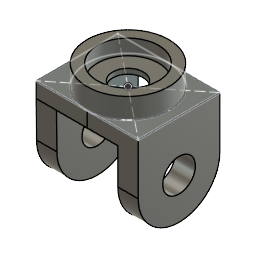
d2 (Autodesk Fusion 360 design; units mm, degrees)
part number: 2026-08-20-16-30-49-448
Autodesk Fusion 360 part; units mm, degrees
sketch "Sketch1" plane through (0, 0, 0) normal (0, 1, 0) x (1, 0, 0)
  line L0 (50, 40) -> (-50, 40)
  line L1 (-50, 40) -> (-50, -40)
  line L2 (-50, -40) -> (50, -40)
  line L3 (50, -40) -> (50, 40)
  line L4 (50, 40) -> (-50, -40) construction
  line L5 (-50, 40) -> (50, -40) construction
  circle A0 centre (0, 0) radius 40
  dimension "d1" = 100
  dimension "d2" = 80
  constraint horizontal L0
  constraint perpendicular L0 L1
  constraint parallel L0 L2
  constraint parallel L1 L3
  constraint coincident L4 A0.centre
  constraint coincident L5 A0.centre
  constraint coincident A0.centre origin
  constraint tangent L0 A0
  measures "d1" distance of L1.end L2.end
  measures "d2" distance of L0.end L1.end
extrude "Extrude1" add sketch "Sketch1" against normal blind 15 contours L0 L2 L3 A0 | L0 L1 L2 A0 makes body 1 at (-3.9827, -10, 39.8012)
extrude "Extrude2" add sketch "Sketch1" along normal blind 20 separate body contours A0 makes body 2
sketch "Sketch2" plane through (0, 20, 0) normal (0, 1, 0) x (-1, 0, 0)
  circle A0 centre (0, 0) radius 40
  circle A1 centre (0, 0) radius 30
  dimension "d7" = 60
  constraint concentric A0 A1
  measures "d7" diameter of A1
extrude "Extrude3" cut sketch "Sketch2" against normal blind 15 contours A1 bodies 2
sketch "Sketch3" plane through (0, 5, 0) normal (0, 1, 0) x (-1, 0, 0)
  circle A0 centre (0, 0) radius 30
  circle A1 centre (0, 0) radius 15
  dimension "d10" = 30
  constraint coincident A0.centre A1.centre
  measures "d10" diameter of A1
extrude "Extrude4" cut sketch "Sketch3" against normal blind 20 contours A1 bodies 2
sketch "Sketch4" plane through (50, 0, 0) normal (1, 0, 0) x (0, 0, -1)
  line L0 (40, 0) -> (-40, 0)
  line L1 (-40, 0) -> (-40, -15)
  line L2 (-40, -15) -> (40, -15)
  line L3 (40, -15) -> (40, 0)
  line L4 (40, -15) -> (40, -50)
  line L5 (-40, -50) -> (-40, -15)
  circle A0 centre (0, -50) radius 16
  arc A1 (-40, -50) -> (40, -50) centre (0, -50) ccw
  line L6 (-40, -15) -> (40, -15)
  dimension "d14" = 80
  dimension "d15" = 32
  dimension "d16" = 50
  constraint vertical L4
  constraint vertical L5
  constraint concentric A0 A1
  constraint coincident L1.end L2.start
  constraint coincident L2.end L3.start
  measures "d14" diameter of A1
  measures "d15" diameter of A0
  measures "d16" distance of A0.centre origin
extrude "Extrude5" add sketch "Sketch4" against normal blind 20 separate body contours L2 L4 L5 A1 L6 makes body 3
sketch "Sketch5" plane through (-50, 0, 0) normal (-1, 0, 0) x (0, 0, 1)
  line L0 (40, 0) -> (-40, 0)
  line L1 (-40, 0) -> (-40, -15)
  line L2 (-40, -15) -> (40, -15)
  line L3 (40, -15) -> (40, 0)
  line L4 (-40, -15) -> (40, -15)
  line L5 (-40, -15) -> (-40, -50)
  arc A0 (-40, -50) -> (0, -90) centre (0, -50) ccw
  arc A1 (0, -90) -> (39.5309, -50.4691) centre (0, -50.4691) ccw
  line L6 (39.5309, -50.4691) -> (40, -15)
  circle A2 centre (0, -50) radius 15
  dimension "d19" = 30
  constraint coincident L1.end L2.start
  constraint coincident L2.end L3.start
  constraint perpendicular L4 L5
  constraint tangent L5 A0
  constraint tangent A0 A1
  constraint concentric A0 A2
  measures "d19" diameter of A2
extrude "Extrude6" add sketch "Sketch5" against normal blind 20 separate body contours L2 L4 L5 A0 A1 L6 makes body 4
combine "Combine1" operation add target body 4 tool bodies 1 3 2
